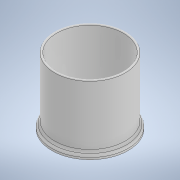
# Autodesk Inventor part: BASE
Saved by Autodesk Inventor 2022 (Build 260153000, 153)
## iProperties
Created: 2022-03-20
Part Number: BASE
Material: Generico
Document SubType Name: Modeling
Designer: dutto
Density: 1 g/cm^3
Appearance: Default
Author: dutto
Autodesk Inventor part; units mm, degrees
ref_plane "YZ Plane" through (0, 0, 0) normal (1, 0, 0) x (0, 1, 0)
ref_plane "XZ Plane" through (0, 0, 0) normal (0, 1, 0) x (-1, 0, 0)
ref_plane "XY Plane" through (0, 0, 0) normal (0, 0, 1) x (1, 0, 0)
sketch "Schizzo1" plane through (0, 0, 0) normal (0, 1, 0) x (-1, 0, 0)
  circle A0 centre (40, -50) radius 40
  point P0 (0, 0)
  constraints: 1 centre point
extrude "Estrusione1" add sketch "Schizzo1" along normal blind 5
fillet "Raccordo1" radius 3 1 edges at (0, 5, -50)
sketch "Schizzo2" plane through (-40, 5, -50) normal (0, 1, 0) x (1, 0, 0)
  circle A0 centre (0, 0) radius 37
  point P0 (40, -50)
  constraints: 1 centre point
extrude "Estrusione2" add sketch "Schizzo2" along normal blind 65
fillet "Raccordo2" radius 3 2 edges at (-40, 5, -87) (-40, 5, -13)
sketch "Schizzo3" plane through (-40, 70, -50) normal (0, 1, 0) x (1, 0, 0)
  circle A0 centre (0, 0) radius 35
  point P0 (40, -50)
  dimension "d8" = 70
  constraints: 1 centre point
  measures "d8" diameter of A0
extrude "Estrusione3" cut sketch "Schizzo3" against normal blind 65
fillet "Raccordo3" radius 1 2 edges at (-75, 70, -50) (-77, 70, -50)
fillet "Raccordo4" radius 3 1 edges at (-75, 5, -50)
